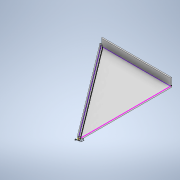
# Autodesk Inventor part: SolarMountLeft
Saved by Autodesk Inventor 2021 (Build 250183000, 183)
## iProperties
Created: 2021-02-26
Part Number: SolarMountLeft
Material: Generisch
Document SubType Name: Modeling
Designer: michox
Density: 1 g/cm^3
Appearance: Vorgabe
Author: michox
Autodesk Inventor part; units mm, degrees
ref_plane "YZ Plane" through (0, 0, 0) normal (1, 0, 0) x (0, 1, 0)
ref_plane "XZ Plane" through (0, 0, 0) normal (0, 1, 0) x (-1, 0, 0)
ref_plane "XY Plane" through (0, 0, 0) normal (0, 0, 1) x (1, 0, 0)
sketch "Skizze1" plane through (0, 0, 0) normal (0, 1, 0) x (-1, 0, 0)
  line L0 (0, 0) -> (198.599, 0)
  line L1 (198.599, 0) -> (0, 263.5497)
  line L2 (0, 263.5497) -> (0, 0)
  line L3 (-198.599, 0) -> (0, -263.5497)
  line L4 (0, 0) -> (-198.599, 0)
  line L5 (-198.599, 0) -> (0, -263.5497)
  line L6 (0, -263.5497) -> (-3.3543, -266.0773)
  line L7 (-3.3543, -266.0773) -> (-201.9532, -2.5276)
  line L8 (-201.9532, -2.5276) -> (-198.599, 0)
  line L9 (-195.878, -3.6109) -> (0, -3.6109)
  line L10 (0, -263.5497) -> (0, 0)
  line L11 (0, -3.6109) -> (0, 0)
  line L12 (-1.6771, -264.8135) -> (-200.2761, -1.2638)
  line L13 (-195.878, -3.6109) -> (-198.599, 0)
  line L14 (0, 0) -> (-198.599, 0)
  line L15 (-1.6771, -264.8135) -> (-3.3543, -266.0773)
  line L16 (0, 263.5497) -> (1.6771, 264.8135)
  line L17 (1.6771, 264.8135) -> (200.2761, 1.2638)
  line L18 (200.2761, 1.2638) -> (198.599, 0)
  line L19 (200.2761, 1.2638) -> (201.9532, 2.5276)
  line L20 (201.9532, 2.5276) -> (3.9544, 265.281)
  line L21 (3.3543, 266.0773) -> (1.6771, 264.8135)
  line L22 (2.3571, 266.0773) -> (1, 266.0773)
  line L23 (0, 265.0773) -> (0, 263.5497)
  arc A0 (3.9544, 265.281) -> (2.3571, 266.0773) centre (2.3571, 264.0773) ccw
  arc A1 (1, 266.0773) -> (0, 265.0773) centre (1, 265.0773) ccw
  point P0 (3.1416, 265.9171)
  dimension "d0" = 37
  dimension "d1" = 330
  dimension "d7" = 4.2
  dimension "d8" = 2.1
  dimension "d9" = 2.1
  dimension "d11" = 2
  dimension "d12" = 1
  constraints: 48 end point, 9 perpendicular, 6 point on line, 4 horizontal, 4 point on circle, 4 tangent, 2 centre point, 2 collinear, 2 midpoint, 1 parallel
  measures "d0" angle of L1 L2
  measures "d1" distance of L0.end L1.end
  measures "d7" distance of L3.end L6.end
  measures "d8" distance of L1.end L16.end
  measures "d9" distance of L17.end L19.end
  measures "d11" radius of A0
  measures "d12" radius of A1
extrude "Extrusion1" add sketch "Skizze1" along normal blind 5 contours L2 L1 L0 | L1 L16 L17 L18 | L23 A1 L22 A0 L21 L16 | L17 L21 A0 L20 L19
sketch "Skizze2" plane through (0, 5, 0) normal (0, 1, 0) x (1, 0, 0)
  line L0 (-198.599, 0) -> (0, -263.5497) projected
  line L1 (0, 0) -> (-198.599, 0)
  line L2 (-198.599, 0) -> (0, -263.5497)
  line L3 (0, -263.5497) -> (-3.1416, -265.9171)
  line L4 (-3.3543, -266.0773) -> (-201.9532, -2.5276)
  line L5 (-201.9532, -2.5276) -> (-198.599, 0)
  line L6 (-195.878, -3.6109) -> (0, -3.6109)
  line L7 (0, -263.5497) -> (0, 0) projected
  line L8 (0, -3.6109) -> (0, 0)
  line L9 (-1.6771, -264.8135) -> (-200.2761, -1.2638)
  line L10 (-195.878, -3.6109) -> (-198.599, 0)
  line L11 (0, 0) -> (-198.599, 0) projected
  line L12 (-1.6771, -264.8135) -> (-3.3543, -266.0773)
  line L13 (-193.2485, -3.6109) -> (0, -260.0603)
  line L14 (0, -260.0603) -> (0, -263.5497)
  line L15 (0, -265.0773) -> (0, 0) projected
  line L16 (0, 0) -> (-198.599, 0) projected
  line L17 (-198.599, 0) -> (-201.9532, -2.5276) projected
  line L18 (-201.9532, -2.5276) -> (-3.9544, -265.281) projected
  arc A0 (-3.9544, -265.281) -> (-2.3571, -266.0773) centre (-2.3571, -264.0773) ccw projected
  line L19 (-2.3571, -266.0773) -> (-1, -266.0773) projected
  arc A1 (-1, -266.0773) -> (0, -265.0773) centre (-1, -265.0773) ccw projected
  line L20 (-3.1416, -265.9171) -> (-3.3543, -266.0773)
  point P0 (-3.9544, -265.281)
  dimension "d4" = 4.2
  dimension "d10" = 2.1
  constraints: 26 end point, 7 point on line, 6 perpendicular, 3 collinear, 2 horizontal, 1 midpoint, 1 parallel, 1 point on circle
  measures "d4" distance of L0.end L4.start
  measures "d10" distance between parallel lines of L13 L0
extrude "Extrusion2" add sketch "Skizze2" along normal blind 5 contours L6 L13 L7 L0 | L9 L3 A0 L4 L5 | L15 A1 L19 A0 L3
extrude "Extrusion3" add sketch "Skizze2" along normal blind 20 contours L1 L7 L6 L0
